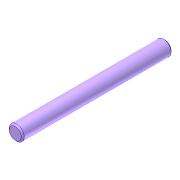
# Autodesk Inventor part: Pin
Saved by Autodesk Inventor 2016 (Build 200138000, 138)
## iProperties
Created: 2010-08-06
Part Number: Pin
Document SubType Name: Modeling
Designer: nguyenducthang
Density: 1 g/cm^3
Mass: 0.00782466 g
Surface Area: 0.325926 cm^2
Volume: 0.00782466 cm^3
Material: Generic
Appearance: Violet
Author: nguyenducthang
Autodesk Inventor part; units mm, degrees
ref_plane "YZ Plane" through (0, 0, 0) normal (1, 0, 0) x (0, 1, 0)
ref_plane "XZ Plane" through (0, 0, 0) normal (0, 1, 0) x (-1, 0, 0)
ref_plane "XY Plane" through (0, 0, 0) normal (0, 0, 1) x (1, 0, 0)
sketch "Sketch47" plane through (0, 0, 0) normal (0, 0, 1) x (1, 0, 0)
  circle A0 centre (0, 0) radius 0.5
  dimension "d264" = 1
  constraints: 1 centre point
  measures "d264" diameter of A0
extrude "Extrusion42" add sketch "Sketch47" along normal blind 10
chamfer "Chamfer6" distance 0.1 angle 45 2 edges at (-0.5, 0, 10) (-0.5, 0, 0)
body "Solid1"
